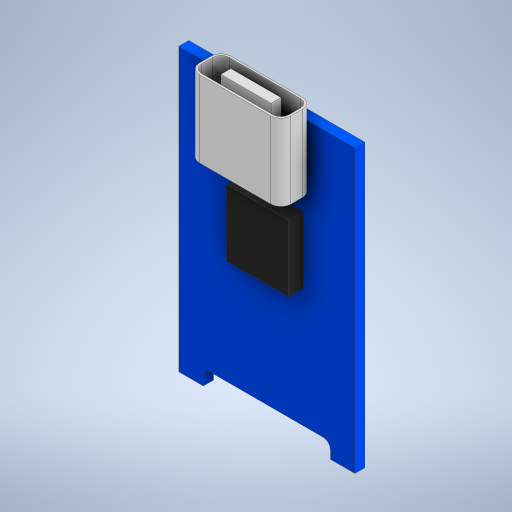
# Autodesk Inventor part: C타입 충전단자
Saved by Autodesk Inventor 2023.1 (Build 271208000, 208)
## iProperties
Created: 2022-08-10
Part Number: C타입 충전단자
Material: 일반
Document SubType Name: Modeling
Designer: fly01
Density: 1 g/cm^3
Appearance: 기본값
Author: fly01
Autodesk Inventor part; units mm, degrees
ref_plane "YZ Plane" through (0, 0, 0) normal (1, 0, 0) x (0, 1, 0)
ref_plane "XZ Plane" through (0, 0, 0) normal (0, 1, 0) x (-1, 0, 0)
ref_plane "XY Plane" through (0, 0, 0) normal (0, 0, 1) x (1, 0, 0)
sketch "스케치1" plane through (0, 0, 0) normal (0, 0, 1) x (1, 0, 0)
  line L0 (-8.75, -14) -> (8.75, -14)
  line L1 (8.75, -14) -> (8.75, 14)
  line L2 (8.75, 14) -> (-8.75, 14)
  line L3 (-8.75, 14) -> (-8.75, -14)
  line L4 (-8.75, -14) -> (8.75, 14) construction
  line L5 (8.75, -14) -> (-8.75, 14) construction
  line L6 (-8.75, -14) -> (-6.31, -14)
  line L7 (-6.31, -14) -> (-6.31, -12.46)
  line L8 (-6.31, -12.46) -> (0, -12.46)
  line L9 (0, 0) -> (0, 2.6603)
  line L10 (8.75, -14) -> (6.31, -14)
  line L11 (6.31, -14) -> (6.31, -12.46)
  line L12 (6.31, -12.46) -> (0, -12.46)
  dimension "d0" = 17.5
  dimension "d1" = 28
  dimension "d2" = 2.44
  dimension "d3" = 1.54
  constraints: 26 end point, 3 perpendicular, 2 midpoint, 2 parallel, 2 symmetric about line, 1 horizontal, 1 point on line, 1 vertical
  measures "d0" distance of L2.end L1.end
  measures "d1" distance of L1.end L0.end
  measures "d2" distance of L0.start L6.end
  measures "d3" distance of L6.end L7.end
extrude "돌출1" add sketch "스케치1" along normal blind 1 contours L3 L2 L1 L0 L11 L12 L8 L7
sketch "스케치2" plane through (-8.75, 14, 0) normal (0, 1, 0) x (1, 0, 0)
  line L0 (5.2, -1) -> (12.3, -1)
  line L1 (13.3, -2) -> (13.3, -3.15)
  line L2 (12.3, -4.15) -> (5.2, -4.15)
  line L3 (4.2, -3.15) -> (4.2, -2)
  line L4 (4.2, -1) -> (13.3, -4.15) construction
  line L5 (13.3, -1) -> (4.2, -4.15) construction
  line L6 (17.5, -1) -> (0, -1) construction
  line L7 (6.25, -2.075) -> (11.25, -2.075)
  line L8 (11.25, -2.075) -> (11.25, -3.075)
  line L9 (11.25, -3.075) -> (6.25, -3.075)
  line L10 (6.25, -3.075) -> (6.25, -2.075)
  line L11 (6.25, -2.075) -> (11.25, -3.075) construction
  line L12 (11.25, -2.075) -> (6.25, -3.075) construction
  arc A0 (13.3, -2) -> (12.3, -1) centre (12.3, -2) ccw
  arc A1 (12.3, -4.15) -> (13.3, -3.15) centre (12.3, -3.15) ccw
  arc A2 (5.2, -1) -> (4.2, -2) centre (5.2, -2) ccw
  arc A3 (4.2, -3.15) -> (5.2, -4.15) centre (5.2, -3.15) ccw
  line L13 (13.1, -3.15) -> (13.1, -2)
  arc A4 (13.1, -2) -> (12.3, -1.2) centre (12.3, -2) ccw
  line L14 (12.3, -1.2) -> (5.2, -1.2)
  arc A5 (5.2, -1.2) -> (4.4, -2) centre (5.2, -2) ccw
  line L15 (4.4, -2) -> (4.4, -3.15)
  arc A6 (4.4, -3.15) -> (5.2, -3.95) centre (5.2, -3.15) ccw
  line L16 (5.2, -3.95) -> (12.3, -3.95)
  arc A7 (12.3, -3.95) -> (13.1, -3.15) centre (12.3, -3.15) ccw
  point P0 (8.75, 0)
  point P1 (8.75, -2.575)
  point P2 (8.75, -1)
  dimension "d6" = 3.15
  dimension "d7" = 9.1
  dimension "d8" = 5
  dimension "d9" = 1
  dimension "d10" = 1
  dimension "d11" = 0.2
  constraints: 32 end point, 16 point on circle, 8 centre point, 8 point on line, 8 tangent, 6 midpoint, 6 parallel, 3 equal radius, 3 perpendicular, 2 horizontal, 7 other
  measures "d6" distance of L5.start L4.end
  measures "d7" distance of L4.end L5.end
  measures "d8" distance of L8.end L9.end
  measures "d9" distance of L7.end L8.end
  measures "d10" radius of A0
  measures "d11" distance between parallel lines of L1 L13
extrude "돌출2" add sketch "스케치2" along normal blind 1.74 and the other way blind 5.86
fillet "모깎기1" radius 0.7 2 edges at (6.31, -12.46, 0.5) (-6.31, -12.46, 0.5)
sketch "스케치3" plane through (-8.75, 8.14, 0) normal (0, -1, 0) x (1, 0, 0)
  line L0 (12.3, 4.15) -> (5.2, 4.15) projected
  arc A0 (5.2, 4.15) -> (4.2, 3.15) centre (5.2, 3.15) ccw projected
  line L1 (4.2, 3.15) -> (4.2, 2) projected
  arc A1 (4.2, 2) -> (5.2, 1) centre (5.2, 2) ccw projected
  line L2 (12.3, 1) -> (5.2, 1) projected
  arc A2 (12.3, 1) -> (13.3, 2) centre (12.3, 2) ccw projected
  line L3 (13.3, 2) -> (13.3, 3.15) projected
  arc A3 (13.3, 3.15) -> (12.3, 4.15) centre (12.3, 3.15) ccw projected
  arc A4 (13.1, 3.15) -> (12.3, 3.95) centre (12.3, 3.15) ccw projected
  line L4 (13.1, 3.15) -> (13.1, 2) projected
  arc A5 (12.3, 1.2) -> (13.1, 2) centre (12.3, 2) ccw projected
  line L5 (12.3, 1.2) -> (5.2, 1.2) projected
  arc A6 (4.4, 2) -> (5.2, 1.2) centre (5.2, 2) ccw projected
  line L6 (4.4, 2) -> (4.4, 3.15) projected
  arc A7 (5.2, 3.95) -> (4.4, 3.15) centre (5.2, 3.15) ccw projected
  line L7 (5.2, 3.95) -> (12.3, 3.95) projected
  point P0 (8.75, 0)
extrude "돌출3" add sketch "스케치3" against normal blind 1 contours A3 L3 A2 L2 A1 L1 A0 L0 | L4 A5 L5 A6 L6 A7 L7 A4
sketch "스케치4" plane through (0, 0, 1) normal (0, 0, 1) x (1, 0, 0)
  line L0 (3.631, 5.9375) -> (-2.5, 5.9375)
  line L1 (-2.5, 5.9375) -> (-2.5, -0.6101)
  line L2 (-2.5, -0.6101) -> (3.631, -0.6101)
  line L3 (3.631, -0.6101) -> (3.631, 5.9375)
  line L4 (3.631, 5.9375) -> (-2.5, -0.6101) construction
  line L5 (-2.5, 5.9375) -> (3.631, -0.6101) construction
  point P0 (0, 0)
  point P1 (0.5655, 2.6637)
  constraints: 12 end point, 2 midpoint, 2 parallel, 1 horizontal, 1 perpendicular
extrude "돌출4" add sketch "스케치4" along normal blind 1.5
